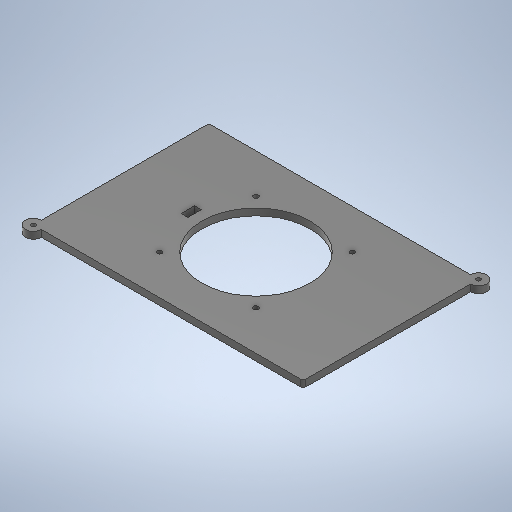
# Autodesk Inventor part: LED Power Box (12V) Cover
Saved by Autodesk Inventor 2026.2 (Build 302298010, 298A)
## iProperties
Created: 2026-05-25
Part Number: LED Power Box (12V) Cover
Material: ABS Plastic
Document SubType Name: Modeling
Designer: chanh
Density: 1.06 g/cm^3
Appearance: Smooth - White
Author: chanh
Autodesk Inventor part; units mm, degrees
ref_plane "YZ Plane" through (0, 0, 0) normal (1, 0, 0) x (0, 1, 0)
ref_plane "XZ Plane" through (0, 0, 0) normal (0, 1, 0) x (-1, 0, 0)
ref_plane "XY Plane" through (0, 0, 0) normal (0, 0, 1) x (1, 0, 0)
sketch "Sketch1" plane through (0, 0, 0) normal (0, 1, 0) x (-1, 0, 0)
  line L0 (100, 65) -> (-100, 65)
  line L1 (-100, 65) -> (-100, -65)
  line L2 (-100, -65) -> (100, -65)
  line L3 (100, -65) -> (100, 65)
  line L4 (100, 65) -> (-100, -65) construction
  line L5 (-100, 65) -> (100, -65) construction
  circle A0 centre (100, 65) radius 6
  circle A1 centre (-100, -65) radius 6
  point P0 (0, 0)
  point P1 (94, 65)
  point P2 (100, 59)
  point P3 (-100, -59)
  point P4 (-94, -65)
  dimension "d0" = 200
  dimension "d1" = 130
  dimension "d4" = 12
  constraints: 12 end point, 2 centre point, 2 coincident, 2 midpoint, 2 parallel, 1 equal radius, 1 horizontal, 1 perpendicular
  measures "d0" distance of L2.end L1.end
  measures "d1" distance of L1.end L0.end
  measures "d4" diameter of A0
extrude "Extrusion1" add sketch "Sketch1" along normal blind 5
fillet "Fillet1" radius 2 2 edges at (100, 2.5, 65) (-100, 2.5, -65)
sketch "Sketch2" plane through (0, 5, 0) normal (0, 1, 0) x (1, 0, 0)
  arc A0 (-98, 65) -> (-100, 63) centre (-98, 63) ccw projected
  line L0 (-100, 63) -> (-100, -59) projected
  arc A1 (-100, -59) -> (-94, -65) centre (-100, -65) ccw projected
  line L1 (-94, -65) -> (98, -65) projected
  arc A2 (98, -65) -> (100, -63) centre (98, -63) ccw projected
  line L2 (100, -63) -> (100, 59) projected
  arc A3 (100, 59) -> (94, 65) centre (100, 65) ccw projected
  line L3 (94, 65) -> (-98, 65) projected
  point P0 (0, 0)
hole "Hole1" at (100, 5, -65) at (-100, 5, 65) direction (0, -1, 0) diameter 3.2 end through all
sketch "Sketch3" plane through (0, 5, 0) normal (0, 1, 0) x (1, 0, 0)
  circle A0 centre (0, 0) radius 40
  dimension "d13" = 80
  constraints: 1 centre point, 1 coincident
  measures "d13" diameter of A0
extrude "Extrusion2" cut sketch "Sketch3" against normal through all
sketch "Sketch4" plane through (0, 5, 0) normal (0, 1, 0) x (1, 0, 0)
  line L0 (-35.75, -35.75) -> (35.75, -35.75) construction
  line L1 (35.75, -35.75) -> (35.75, 35.75) construction
  line L2 (35.75, 35.75) -> (-35.75, 35.75) construction
  line L3 (-35.75, 35.75) -> (-35.75, -35.75) construction
  line L4 (-35.75, -35.75) -> (35.75, 35.75) construction
  line L5 (35.75, -35.75) -> (-35.75, 35.75) construction
  point P0 (0, 0)
  dimension "d16" = 71.5
  constraints: 12 end point, 4 coincident, 2 midpoint, 2 parallel, 2 perpendicular, 1 horizontal
  measures "d16" distance of L2.end L1.end
hole "Hole2" at (-35.75, 5, -35.75) at (-35.75, 5, 35.75) at (35.75, 5, 35.75) at (35.75, 5, -35.75) direction (0, -1, 0) diameter 3.7 end through all
sketch "Sketch5" plane through (0, 5, 0) normal (0, 1, 0) x (1, 0, 0)
  line L0 (-52.5, 7) -> (-47.5, 7)
  line L1 (-47.5, 7) -> (-47.5, -3)
  line L2 (-47.5, -3) -> (-52.5, -3)
  line L3 (-52.5, -3) -> (-52.5, 7)
  line L4 (-52.5, 7) -> (-47.5, -3) construction
  line L5 (-47.5, 7) -> (-52.5, -3) construction
  line L6 (-100, 63) -> (-100, -59) projected
  point P0 (0, 0)
  point P1 (-50, 2)
  point P2 (-100, 2)
  point P3 (-100, 2)
  dimension "d24" = 50
  dimension "d25" = 5
  dimension "d26" = 10
  constraints: 12 end point, 4 midpoint, 2 parallel, 1 horizontal, 1 horizontal alignment, 1 perpendicular
  measures "d24" distance of point (-100, 2) point (-50, 2)
  measures "d25" distance between parallel lines of L3 L1
  measures "d26" distance of L0.end L1.end
extrude "Extrusion3" cut sketch "Sketch5" against normal through all
body "Solid1"
